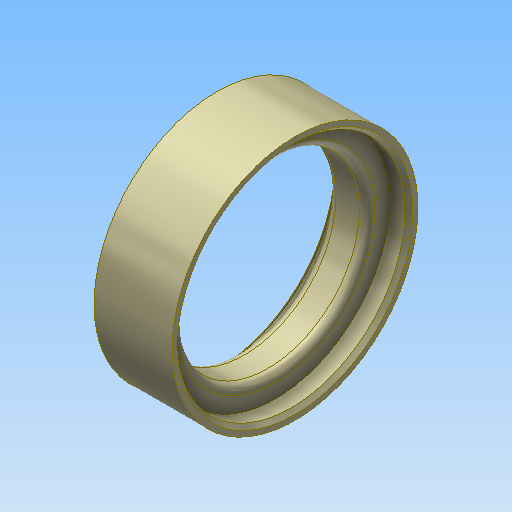
# Autodesk Inventor part: Plunger_Seal
Saved by Autodesk Inventor 2020.1 (Build 241239000, 239)
## iProperties
Created: 2001-02-20
Part Number: Plunger_Seal
Document SubType Name: Modeling
Designer: Joe M
Material: Nylon-6/6
Description: Piston
Engineer: Joe M
Density: 1.13 g/cm^3
Appearance: Nylon 6
Control State: 0
Master: False
Checked Out: False
Shininess: 31.0
Length Units: 11269
Angle Units: 11279
Time Units: 11290
Mass Units: 11283
Length Display Precision: 3
Angle Display Precision: 2
Compacted: True
Density: 1.13
Volumn: 32.42050770303565
Area: 142.99987053837322
PropertySet Name: Model Information
Title: Kolvtätning
Author: Joe M
Autodesk Inventor part; units mm, degrees
ref_plane "YZ Plane" through (0, 0, 0) normal (1, 0, 0) x (0, 1, 0)
ref_plane "XZ Plane" through (0, 0, 0) normal (0, 1, 0) x (-1, 0, 0)
ref_plane "XY Plane" through (0, 0, 0) normal (0, 0, 1) x (1, 0, 0)
sketch "Sketch1" plane through (0, 0, 0) normal (0, 0, 1) x (1, 0, 0)
  line L0 (0, 23.5) -> (3, 23.5)
  line L1 (5, 25.5) -> (5, 29.2)
  line L2 (5, 29.2) -> (10, 29.2)
  line L3 (10, 29.2) -> (10, 31.5)
  line L4 (10, 31.5) -> (0, 31.5)
  line L5 (0, 23.5) -> (0, 39.7331)
  arc A0 (3, 23.5) -> (5, 25.5) centre (3, 25.5) ccw
  line L6 (0, 0) -> (48.7382, 0)
  line L7 (0, 23.5) -> (-3, 23.5)
  line L8 (-5, 25.5) -> (-5, 29.2)
  line L9 (-5, 29.2) -> (-10, 29.2)
  line L10 (-10, 29.2) -> (-10, 31.5)
  line L11 (-10, 31.5) -> (0, 31.5)
  arc A1 (-5, 25.5) -> (-3, 23.5) centre (-3, 25.5) ccw
  dimension "d0" = 2
  dimension "d1" = 47
  dimension "d2" = 63
  dimension "d3" = 58.4
  dimension "d4" = 10
  dimension "d7" = 10
  constraints: 24 end point, 6 symmetric about line, 4 perpendicular, 4 point on circle, 3 parallel, 2 centre point, 2 tangent, 1 coincident, 1 horizontal, 1 point on line, 1 vertical alignment, 6 other
  measures "d0" radius of A0
  measures "d1" diameter of L0 L6
  measures "d2" diameter of L4 L6
  measures "d3" diameter of L2 L6
  measures "d4" distance of L3.end L4.end
  measures "d7" distance between parallel lines of L1 L8
revolve "Revolution1" add sketch "Sketch1" angle 360 about axis through (0, 0, 0) along (1, 0, 0)
chamfer "Fase1" distance 1 angle 45 1 edges at (10, -29.2, 0)
chamfer "Fase2" distance 1 angle 45 1 edges at (-10, -29.2, 0)
body "Solid1"
